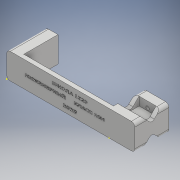
# Autodesk Inventor part: Сбрасывание
Saved by Autodesk Inventor 2018 (Build 220112000, 112)
## iProperties
Created: 2023-02-08
Part Number: Сбрасывание
Material: Типовые
Document SubType Name: Modeling
Designer: exper
Density: 1 g/cm^3
Appearance: По умолчанию
Author: exper
## iProperties of the stored document Сбрасывание_3DПЕЧАТЬ.ipt
Created: 2023-02-08
Part Number: Сбрасывание_3DПЕЧАТЬ
Material: Типовые
Document SubType Name: Modeling
Designer: exper
Density: 1 g/cm^3
Appearance: По умолчанию
Author: exper
Autodesk Inventor part; units mm, degrees
ref_plane "YZ Plane" through (0, 0, 0) normal (1, 0, 0) x (0, 1, 0)
ref_plane "XZ Plane" through (0, 0, 0) normal (0, 1, 0) x (-1, 0, 0)
ref_plane "XY Plane" through (0, 0, 0) normal (0, 0, 1) x (1, 0, 0)
sketch "Эскиз1" plane through (0, 0, 0) normal (0, 0, 1) x (1, 0, 0)
  line L0 (0, 0) -> (150, 0)
  line L1 (0, 0) -> (0, 45)
  line L2 (0, 45) -> (15, 45)
  line L3 (15, 45) -> (15, 5)
  line L4 (150, 0) -> (150, 40)
  line L5 (150, 40) -> (120, 40)
  line L6 (120, 40) -> (120, 5)
  line L7 (120, 5) -> (15, 5)
  dimension "d0" = 150
  dimension "d1" = 45
  dimension "d2" = 15
  dimension "d3" = 40
  dimension "d4" = 40
  dimension "d5" = 30
  dimension "d6" = 35
  constraints: 16 end point, 4 perpendicular, 2 vertical, 1 horizontal
  measures "d0" distance of L0.start L0.end
  measures "d1" distance of L0.start L1.end
  measures "d2" distance of L1.end L2.end
  measures "d3" distance of L2.end L3.end
  measures "d4" distance of L0.end L4.end
  measures "d5" distance of L4.end L5.end
  measures "d6" distance of L5.end L6.end
extrude "Выдавливание1" add sketch "Эскиз1" along normal blind 30
sketch "Эскиз2" plane through (120, 40, 0) normal (0, 1, 0) x (1, 0, 0)
  line L0 (0, 0) -> (0, -30) projected
  point P0 (-120, 0)
  point P1 (15, -15)
  point P2 (15, -15)
  point P3 (15, -15)
  point P4 (15, -7)
  point P5 (15, -23)
  constraints: 2 coincident
hole "Отверстие1" at (135, 40, 15) at (135, 40, 7) at (135, 40, 23) direction (0, -1, 0) diameter 4 depth 20
sketch "Эскиз3" plane through (120, 5, 0) normal (-1, 0, 0) x (0, 0, 1)
  point P0 (0, -5)
sketch "Эскиз4" plane through (120, 40, 0) normal (0, 1, 0) x (1, 0, 0)
  point P0 (-120, 0)
sketch "Эскиз5" plane through (150, 0, 0) normal (1, 0, 0) x (0, 0, -1)
  line L0 (0, 30) -> (-10, 30)
  line L1 (-10, 30) -> (-10, 10)
  line L2 (-10, 10) -> (0, 10)
  line L3 (0, 40) -> (0, 5) projected
  point P0 (0, 0)
  dimension "d19" = 10
  dimension "d20" = 20
  constraints: 6 end point, 1 horizontal, 1 perpendicular, 1 point on line, 1 vertical
  measures "d19" distance of L0.start L0.end
  measures "d20" distance of L0.end L1.end
extrude "Выдавливание2" cut sketch "Эскиз5" against normal blind 30
sketch "Эскиз6" plane through (150, 0, 30) normal (1, 0, 0) x (0, 0, -1)
  line L0 (0, 30) -> (10, 30)
  line L1 (10, 30) -> (10, 10)
  line L2 (10, 10) -> (0, 10)
  line L3 (0, 30) -> (0, 10)
  line L4 (0, 0) -> (0, 40) projected
  point P0 (30, 0)
  dimension "d24" = 10
  constraints: 8 end point, 2 perpendicular, 1 collinear, 1 horizontal
  measures "d24" distance of L0.start L0.end
extrude "Выдавливание3" cut sketch "Эскиз6" against normal blind 30
sketch "Эскиз7" plane through (150, 0, 30) normal (1, 0, 0) x (0, 0, -1)
  line L0 (30, 30) -> (20, 30) projected
  line L1 (30, 30) -> (20, 20)
  line L2 (20, 30) -> (20, 10) projected
  line L3 (30, 10) -> (30, 5) projected
  line L4 (20, 20) -> (30, 10)
  line L5 (30, 10) -> (20, 10)
  line L6 (0, 45) -> (0, 0) projected
  line L7 (20, 20) -> (20, 30)
  point P0 (30, 0)
  constraints: 8 end point, 2 perpendicular, 1 midpoint
extrude "Выдавливание4" add sketch "Эскиз7" against normal blind 5
sketch "Эскиз8" plane through (150, 0, 30) normal (1, 0, 0) x (0, 0, -1)
  line L0 (0, 30) -> (10, 30) projected
  line L1 (0, 30) -> (10, 20)
  line L2 (10, 30) -> (10, 10) projected
  line L3 (10, 10) -> (0, 10) projected
  line L4 (0, 10) -> (10, 20)
  line L5 (10, 10) -> (10, 20)
  line L6 (10, 30) -> (0, 30)
  point P0 (30, 0)
  constraints: 8 end point, 2 perpendicular, 1 midpoint, 1 point on line, 1 vertical
extrude "Выдавливание5" add sketch "Эскиз8" against normal blind 5
sketch "Эскиз9" plane through (120, 40, 0) normal (-1, 0, 0) x (0, 0, 1)
  line L0 (0, -10) -> (10, -10) projected
  line L1 (0, -10) -> (10, -20)
  line L2 (10, -10) -> (10, -30) projected
  line L3 (10, -30) -> (0, -30) projected
  line L4 (0, -30) -> (10, -20)
  line L5 (10, -30) -> (10, -20)
  line L6 (10, -10) -> (0, -10)
  point P0 (0, -40)
  constraints: 8 end point, 2 perpendicular, 1 midpoint, 1 point on line, 1 vertical
extrude "Выдавливание6" add sketch "Эскиз9" against normal blind 5
sketch "Эскиз10" plane through (120, 40, 0) normal (-1, 0, 0) x (0, 0, 1)
  line L0 (30, 0) -> (30, -10) projected
  line L1 (30, -10) -> (20, -20)
  line L2 (20, -30) -> (20, -10) projected
  line L3 (30, -30) -> (20, -30) projected
  line L4 (30, -30) -> (20, -20)
  line L5 (20, -30) -> (20, -20)
  line L6 (20, -10) -> (30, -10) projected
  line L7 (20, -10) -> (30, -10)
  point P0 (0, -40)
  constraints: 8 end point, 1 collinear, 1 midpoint, 1 perpendicular, 1 point on line, 1 vertical
extrude "Выдавливание7" add sketch "Эскиз10" against normal blind 5 contours L4 L3 L2
sketch "Эскиз11" plane through (120, 40, 0) normal (-1, 0, 0) x (0, 0, 1)
  line L0 (20, -10) -> (30, -10) projected
  line L1 (30, -10) -> (20, -20)
  line L2 (20, -20) -> (20, -10) projected
  line L3 (20, -20) -> (20, -10)
  line L4 (20, -10) -> (30, -10)
  point P0 (0, -40)
  constraints: 6 end point, 1 collinear, 1 perpendicular
extrude "Выдавливание8" add sketch "Эскиз11" against normal blind 5
sketch "Эскиз12" plane through (0, 0, 0) normal (0, -1, 0) x (1, 0, 0)
  line L0 (52.9376, 24.6029) -> (106.7977, 24.6029) construction
  line L1 (106.7977, 24.6029) -> (106.7977, 18.3352) construction
  line L2 (106.7977, 18.3352) -> (52.9376, 18.3352) construction
  line L3 (52.9376, 18.3352) -> (52.9376, 24.6029) construction
  line L4 (21.416, 17.5304) -> (72.5083, 17.5304) construction
  line L5 (72.5083, 17.5304) -> (72.5083, 13.5043) construction
  line L6 (72.5083, 13.5043) -> (21.416, 13.5043) construction
  line L7 (21.416, 13.5043) -> (21.416, 17.5304) construction
  line L8 (78.5854, 16.8541) -> (114.6972, 16.8541) construction
  line L9 (114.6972, 16.8541) -> (114.6972, 13.7301) construction
  line L10 (114.6972, 13.7301) -> (78.5854, 13.7301) construction
  line L11 (78.5854, 13.7301) -> (78.5854, 16.8541) construction
  line L12 (25.7653, 13.5409) -> (24.6543, 13.5409)
  line L13 (24.6543, 13.5409) -> (24.6543, 15.5174)
  line L14 (24.6543, 15.5174) -> (22.9258, 13.5409)
  line L15 (22.9258, 13.5409) -> (21.8804, 13.5409)
  line L16 (21.8804, 13.5409) -> (21.8804, 16.5409)
  line L17 (21.8804, 16.5409) -> (22.9914, 16.5409)
  line L18 (22.9914, 16.5409) -> (22.9914, 14.7541)
  line L19 (22.9914, 14.7541) -> (24.5911, 16.5409)
  line L20 (24.5911, 16.5409) -> (25.7653, 16.5409)
  line L21 (25.7653, 16.5409) -> (25.7653, 13.5409)
  line L22 (30.4768, 13.5409) -> (29.3464, 13.5409)
  line L23 (29.3464, 13.5409) -> (29.3464, 14.8708)
  line L24 (29.3464, 14.8708) -> (27.8075, 14.8708)
  line L25 (27.8075, 14.8708) -> (27.8075, 13.5409)
  line L26 (27.8075, 13.5409) -> (26.677, 13.5409)
  line L27 (26.677, 13.5409) -> (26.677, 16.5409)
  line L28 (26.677, 16.5409) -> (27.8075, 16.5409)
  line L29 (27.8075, 16.5409) -> (27.8075, 15.4421)
  line L30 (27.8075, 15.4421) -> (29.3464, 15.4421)
  line L31 (29.3464, 15.4421) -> (29.3464, 16.5409)
  line L32 (29.3464, 16.5409) -> (30.4768, 16.5409)
  line L33 (30.4768, 16.5409) -> (30.4768, 13.5409)
  line L34 (37.4517, 13.5409) -> (36.1219, 13.5409)
  line L35 (36.1219, 13.5409) -> (35.023, 14.7735)
  line L36 (35.023, 14.7735) -> (34.7289, 14.7735)
  line L37 (34.7289, 14.7735) -> (34.7289, 13.5409)
  line L38 (34.7289, 13.5409) -> (33.6057, 13.5409)
  line L39 (33.6057, 13.5409) -> (33.6057, 14.7735)
  line L40 (33.6057, 14.7735) -> (33.2994, 14.7735)
  line L41 (33.2994, 14.7735) -> (32.2005, 13.5409)
  line L42 (32.2005, 13.5409) -> (30.8828, 13.5409)
  line L43 (30.8828, 13.5409) -> (32.2904, 15.0701)
  spline S0 degree 2 poles (32.2904, 15.0701) (32.1859, 15.1114) (31.9987, 15.3108) (31.9015, 15.4907) knots 0 0 0 1 2 2 2
  spline S1 degree 2 poles (31.9015, 15.4907) (31.7872, 15.7095) (31.5173, 15.8894) (31.3083, 15.8894) knots 0 0 0 1 2 2 2
  line L44 (31.3083, 15.8894) -> (31.1041, 15.8894)
  line L45 (31.1041, 15.8894) -> (31.1041, 16.5409)
  spline S2 degree 2 poles (31.1041, 16.5409) (31.1575, 16.5409) (31.3812, 16.5458) (31.5246, 16.5458) knots 0 0 0 1 2 2 2
  spline S3 degree 2 poles (31.5246, 16.5458) (31.9841, 16.5458) (32.5384, 16.3075) (32.711, 16.0426) knots 0 0 0 1 2 2 2
  spline S4 degree 2 poles (32.711, 16.0426) (32.7645, 15.9599) (32.8593, 15.78) (32.9177, 15.6973) knots 0 0 0 1 2 2 2
  spline S5 degree 2 poles (32.9177, 15.6973) (33.0806, 15.4591) (33.3674, 15.2962) (33.6057, 15.2962) knots 0 0 0 1 2 2 2
  line L46 (33.6057, 15.2962) -> (33.6057, 16.5409)
  line L47 (33.6057, 16.5409) -> (34.7289, 16.5409)
  line L48 (34.7289, 16.5409) -> (34.7289, 15.2962)
  spline S6 degree 2 poles (34.7289, 15.2962) (34.9865, 15.2986) (35.2515, 15.4518) (35.4169, 15.6973) knots 0 0 0 1 2 2 2
  spline S7 degree 2 poles (35.4169, 15.6973) (35.4655, 15.7727) (35.5749, 15.9648) (35.6235, 16.0426) knots 0 0 0 1 2 2 2
  spline S8 degree 2 poles (35.6235, 16.0426) (35.7912, 16.3075) (36.348, 16.5458) (36.8099, 16.5458) knots 0 0 0 1 2 2 2
  spline S9 degree 2 poles (36.8099, 16.5458) (36.9655, 16.5458) (37.1721, 16.5409) (37.2305, 16.5409) knots 0 0 0 1 2 2 2
  line L49 (37.2305, 16.5409) -> (37.2305, 15.8967)
  line L50 (37.2305, 15.8967) -> (37.0263, 15.8967)
  spline S10 degree 2 poles (37.0263, 15.8967) (36.7783, 15.8967) (36.5571, 15.7216) (36.4233, 15.5028) knots 0 0 0 1 2 2 2
  spline S11 degree 2 poles (36.4233, 15.5028) (36.3091, 15.3108) (36.1438, 15.1212) (36.0344, 15.0774) knots 0 0 0 1 2 2 2
  line L51 (36.0344, 15.0774) -> (37.4517, 13.5409)
  line L52 (37.8601, 13.5409) -> (37.8601, 16.5409)
  line L53 (37.8601, 16.5409) -> (40.9039, 16.5409)
  line L54 (40.9039, 16.5409) -> (40.9039, 15.9696)
  line L55 (40.9039, 15.9696) -> (38.9833, 15.9696)
  line L56 (38.9833, 15.9696) -> (38.9833, 15.4421)
  line L57 (38.9833, 15.4421) -> (40.7532, 15.4421)
  line L58 (40.7532, 15.4421) -> (40.7532, 14.8708)
  line L59 (40.7532, 14.8708) -> (38.9833, 14.8708)
  line L60 (38.9833, 14.8708) -> (38.9833, 14.1122)
  line L61 (38.9833, 14.1122) -> (40.9039, 14.1122)
  line L62 (40.9039, 14.1122) -> (40.9039, 13.5409)
  line L63 (40.9039, 13.5409) -> (37.8601, 13.5409)
  line L64 (45.4671, 13.5409) -> (44.3366, 13.5409)
  line L65 (44.3366, 13.5409) -> (44.3366, 14.8708)
  line L66 (44.3366, 14.8708) -> (42.7977, 14.8708)
  line L67 (42.7977, 14.8708) -> (42.7977, 13.5409)
  line L68 (42.7977, 13.5409) -> (41.6673, 13.5409)
  line L69 (41.6673, 13.5409) -> (41.6673, 16.5409)
  line L70 (41.6673, 16.5409) -> (42.7977, 16.5409)
  line L71 (42.7977, 16.5409) -> (42.7977, 15.4421)
  line L72 (42.7977, 15.4421) -> (44.3366, 15.4421)
  line L73 (44.3366, 15.4421) -> (44.3366, 16.5409)
  line L74 (44.3366, 16.5409) -> (45.4671, 16.5409)
  line L75 (45.4671, 16.5409) -> (45.4671, 13.5409)
  line L76 (46.3934, 13.5409) -> (46.3934, 16.5409)
  line L77 (46.3934, 16.5409) -> (49.4371, 16.5409)
  line L78 (49.4371, 16.5409) -> (49.4371, 15.9696)
  line L79 (49.4371, 15.9696) -> (47.5165, 15.9696)
  line L80 (47.5165, 15.9696) -> (47.5165, 15.4421)
  line L81 (47.5165, 15.4421) -> (49.2864, 15.4421)
  line L82 (49.2864, 15.4421) -> (49.2864, 14.8708)
  line L83 (49.2864, 14.8708) -> (47.5165, 14.8708)
  line L84 (47.5165, 14.8708) -> (47.5165, 14.1122)
  line L85 (47.5165, 14.1122) -> (49.4371, 14.1122)
  line L86 (49.4371, 14.1122) -> (49.4371, 13.5409)
  line L87 (49.4371, 13.5409) -> (46.3934, 13.5409)
  spline S12 degree 2 poles (53.6648, 15.5952) (53.6648, 15.3861) (53.4655, 15.0069) (53.2783, 14.8805) knots 0 0 0 1 2 2 2
  spline S13 degree 2 poles (53.2783, 14.8805) (53.164, 14.8003) (52.8869, 14.669) (52.7216, 14.6228) knots 0 0 0 1 2 2 2
  spline S14 degree 2 poles (52.7216, 14.6228) (52.5562, 14.5766) (52.1648, 14.5231) (51.9242, 14.5231) knots 0 0 0 1 2 2 2
  line L88 (51.9242, 14.5231) -> (51.331, 14.5231)
  line L89 (51.331, 14.5231) -> (51.331, 13.5409)
  line L90 (51.331, 13.5409) -> (50.2005, 13.5409)
  line L91 (50.2005, 13.5409) -> (50.2005, 16.5409)
  line L92 (50.2005, 16.5409) -> (51.9485, 16.5409)
  spline S15 degree 2 poles (51.9485, 16.5409) (52.3374, 16.5409) (52.9039, 16.4461) (53.1324, 16.344) knots 0 0 0 1 2 2 2
  spline S16 degree 2 poles (53.1324, 16.344) (53.3877, 16.2297) (53.6648, 15.8554) (53.6648, 15.5952) knots 0 0 0 1 2 2 2
  spline S17 degree 2 poles (52.5052, 15.5758) (52.5052, 15.7046) (52.3229, 15.887) (52.1964, 15.921) knots 0 0 0 1 2 2 2
  spline S18 degree 2 poles (52.1964, 15.921) (52.036, 15.9672) (51.7418, 15.9818) (51.4914, 15.9818) knots 0 0 0 1 2 2 2
  line L93 (51.4914, 15.9818) -> (51.331, 15.9818)
  line L94 (51.331, 15.9818) -> (51.331, 15.0823)
  line L95 (51.331, 15.0823) -> (51.4088, 15.0823)
  spline S19 degree 2 poles (51.4088, 15.0823) (51.5692, 15.0823) (51.8536, 15.0871) (51.9606, 15.0993) knots 0 0 0 1 2 2 2
  spline S20 degree 2 poles (51.9606, 15.0993) (52.0506, 15.109) (52.2548, 15.1673) (52.3083, 15.2038) knots 0 0 0 1 2 2 2
  spline S21 degree 2 poles (52.3083, 15.2038) (52.4225, 15.2767) (52.5052, 15.4396) (52.5052, 15.5758) knots 0 0 0 1 2 2 2
  line L96 (58.0652, 13.5409) -> (56.9347, 13.5409)
  line L97 (56.9347, 13.5409) -> (56.9347, 14.8708)
  line L98 (56.9347, 14.8708) -> (55.3958, 14.8708)
  line L99 (55.3958, 14.8708) -> (55.3958, 13.5409)
  line L100 (55.3958, 13.5409) -> (54.2653, 13.5409)
  line L101 (54.2653, 13.5409) -> (54.2653, 16.5409)
  line L102 (54.2653, 16.5409) -> (55.3958, 16.5409)
  line L103 (55.3958, 16.5409) -> (55.3958, 15.4421)
  line L104 (55.3958, 15.4421) -> (56.9347, 15.4421)
  line L105 (56.9347, 15.4421) -> (56.9347, 16.5409)
  line L106 (56.9347, 16.5409) -> (58.0652, 16.5409)
  line L107 (58.0652, 16.5409) -> (58.0652, 13.5409)
  spline S22 degree 2 poles (62.5384, 14.5012) (62.5384, 14.28) (62.288, 13.9129) (62.0692, 13.7938) knots 0 0 0 1 2 2 2
  spline S23 degree 2 poles (62.0692, 13.7938) (61.8115, 13.6552) (61.2086, 13.5409) (60.7759, 13.5409) knots 0 0 0 1 2 2 2
  line L108 (60.7759, 13.5409) -> (58.9914, 13.5409)
  line L109 (58.9914, 13.5409) -> (58.9914, 16.5409)
  line L110 (58.9914, 16.5409) -> (60.1195, 16.5409)
  line L111 (60.1195, 16.5409) -> (60.1195, 15.4153)
  line L112 (60.1195, 15.4153) -> (60.7953, 15.4153)
  spline S24 degree 2 poles (60.7953, 15.4153) (61.1916, 15.4153) (61.831, 15.34) (62.0935, 15.2038) knots 0 0 0 1 2 2 2
  spline S25 degree 2 poles (62.0935, 15.2038) (62.3269, 15.0823) (62.5384, 14.7176) (62.5384, 14.5012) knots 0 0 0 1 2 2 2
  line L113 (64.0044, 13.5409) -> (62.8739, 13.5409)
  line L114 (62.8739, 13.5409) -> (62.8739, 16.5409)
  line L115 (62.8739, 16.5409) -> (64.0044, 16.5409)
  line L116 (64.0044, 16.5409) -> (64.0044, 13.5409)
  spline S26 degree 2 poles (61.3715, 14.4793) (61.3715, 14.5523) (61.3229, 14.686) (61.2426, 14.7419) knots 0 0 0 1 2 2 2
  spline S27 degree 2 poles (61.2426, 14.7419) (61.16, 14.7978) (60.8755, 14.861) (60.6251, 14.861) knots 0 0 0 1 2 2 2
  line L117 (60.6251, 14.861) -> (60.1195, 14.861)
  line L118 (60.1195, 14.861) -> (60.1195, 14.0977)
  line L119 (60.1195, 14.0977) -> (60.6251, 14.0977)
  spline S28 degree 2 poles (60.6251, 14.0977) (60.9703, 14.0977) (61.3715, 14.2921) (61.3715, 14.4793) knots 0 0 0 1 2 2 2
  line L120 (68.818, 13.5409) -> (67.707, 13.5409)
  line L121 (67.707, 13.5409) -> (67.707, 15.5174)
  line L122 (67.707, 15.5174) -> (65.9784, 13.5409)
  line L123 (65.9784, 13.5409) -> (64.9331, 13.5409)
  line L124 (64.9331, 13.5409) -> (64.9331, 16.5409)
  line L125 (64.9331, 16.5409) -> (66.0441, 16.5409)
  line L126 (66.0441, 16.5409) -> (66.0441, 14.7541)
  line L127 (66.0441, 14.7541) -> (67.6438, 16.5409)
  line L128 (67.6438, 16.5409) -> (68.818, 16.5409)
  line L129 (68.818, 16.5409) -> (68.818, 13.5409)
  spline S29 degree 2 poles (68.4776, 17.5304) (68.4752, 17.1682) (67.6972, 16.733) (66.8828, 16.733) knots 0 0 0 1 2 2 2
  spline S30 degree 2 poles (66.8828, 16.733) (66.0806, 16.733) (65.288, 17.173) (65.2856, 17.5304) knots 0 0 0 1 2 2 2
  line L130 (65.2856, 17.5304) -> (66.2775, 17.5304)
  spline S31 degree 2 poles (66.2775, 17.5304) (66.2823, 17.3116) (66.5498, 17.1122) (66.8828, 17.1122) knots 0 0 0 1 2 2 2
  spline S32 degree 2 poles (66.8828, 17.1122) (67.2135, 17.1122) (67.4809, 17.314) (67.4857, 17.5304) knots 0 0 0 1 2 2 2
  line L131 (67.4857, 17.5304) -> (68.4776, 17.5304)
  line L132 (53.5096, 24.5589) -> (54.3074, 24.5589)
  line L133 (54.3074, 24.5589) -> (54.369, 24.5149)
  line L134 (54.369, 24.5149) -> (54.369, 21.8781)
  line L135 (54.369, 21.8781) -> (55.8032, 21.8781)
  line L136 (55.8032, 21.8781) -> (55.8032, 24.5149)
  line L137 (55.8032, 24.5149) -> (55.8678, 24.5589)
  line L138 (55.8678, 24.5589) -> (56.6568, 24.5589)
  line L139 (56.6568, 24.5589) -> (56.7184, 24.5149)
  line L140 (56.7184, 24.5149) -> (56.7184, 21.8781)
  line L141 (56.7184, 21.8781) -> (58.1263, 21.8781)
  line L142 (58.1263, 21.8781) -> (58.1263, 24.5149)
  line L143 (58.1263, 24.5149) -> (58.1908, 24.5589)
  line L144 (58.1908, 24.5589) -> (58.9798, 24.5589)
  line L145 (58.9798, 24.5589) -> (59.0414, 24.5149)
  line L146 (59.0414, 24.5149) -> (59.0414, 21.4029)
  line L147 (59.0414, 21.4029) -> (58.9798, 21.3589)
  line L148 (58.9798, 21.3589) -> (53.5096, 21.3589)
  line L149 (53.5096, 21.3589) -> (53.4538, 21.4029)
  line L150 (53.4538, 21.4029) -> (53.4538, 24.5149)
  line L151 (53.4538, 24.5149) -> (53.5096, 24.5589)
  line L152 (60.9831, 23.2508) -> (61.467, 23.2508)
  line L153 (61.467, 23.2508) -> (62.6139, 24.5589)
  line L154 (62.6139, 24.5589) -> (63.5437, 24.5589)
  line L155 (63.5437, 24.5589) -> (63.5906, 24.5149)
  line L156 (63.5906, 24.5149) -> (62.2032, 23.0337)
  line L157 (62.2032, 23.0337) -> (63.705, 21.4029)
  line L158 (63.705, 21.4029) -> (63.661, 21.3589)
  line L159 (63.661, 21.3589) -> (62.6755, 21.3589)
  line L160 (62.6755, 21.3589) -> (61.4876, 22.7316)
  line L161 (61.4876, 22.7316) -> (60.9831, 22.7316)
  line L162 (60.9831, 22.7316) -> (60.9831, 21.4029)
  line L163 (60.9831, 21.4029) -> (60.9156, 21.3589)
  line L164 (60.9156, 21.3589) -> (60.1384, 21.3589)
  line L165 (60.1384, 21.3589) -> (60.068, 21.4029)
  line L166 (60.068, 21.4029) -> (60.068, 24.5149)
  line L167 (60.068, 24.5149) -> (60.1384, 24.5589)
  line L168 (60.1384, 24.5589) -> (60.9156, 24.5589)
  line L169 (60.9156, 24.5589) -> (60.9831, 24.5149)
  line L170 (60.9831, 24.5149) -> (60.9831, 23.2508)
  spline S33 degree 2 poles (64.0335, 22.9956) (64.0335, 23.3505) (64.2828, 23.943) (64.799, 24.3683) (65.5998, 24.6029) (66.1512, 24.6029) knots 0 0 0 1 2 3 4 4 4
  line L171 (66.1512, 24.6029) -> (66.2538, 24.6029)
  spline S34 degree 2 poles (66.2538, 24.6029) (66.8053, 24.6029) (67.6089, 24.3683) (68.1252, 23.943) (68.3745, 23.3505) (68.3745, 22.9956) knots 0 0 0 1 2 3 4 4 4
  line L172 (68.3745, 22.9956) -> (68.3745, 22.9076)
  spline S35 degree 2 poles (68.3745, 22.9076) (68.3745, 22.5498) (68.1252, 21.9631) (67.6089, 21.5466) (66.8053, 21.3149) (66.2538, 21.3149) knots 0 0 0 1 2 3 4 4 4
  line L173 (66.2538, 21.3149) -> (66.1512, 21.3149)
  spline S36 degree 2 poles (66.1512, 21.3149) (65.5998, 21.3149) (64.799, 21.5466) (64.2828, 21.9631) (64.0335, 22.5498) (64.0335, 22.9076) knots 0 0 0 1 2 3 4 4 4
  line L174 (64.0335, 22.9076) -> (64.0335, 22.9956)
  spline S37 degree 2 poles (66.1512, 24.0926) (65.8051, 24.0926) (65.3593, 23.94) (65.0923, 23.6555) (64.9867, 23.2478) (64.9867, 22.9956) knots 0 0 0 1 2 3 4 4 4
  line L175 (64.9867, 22.9956) -> (64.9867, 22.9076)
  spline S38 degree 2 poles (64.9867, 22.9076) (64.9867, 22.6553) (65.0923, 22.2564) (65.3593, 21.9749) (65.8051, 21.8253) (66.1512, 21.8253) knots 0 0 0 1 2 3 4 4 4
  line L176 (66.1512, 21.8253) -> (66.2538, 21.8253)
  spline S39 degree 2 poles (66.2538, 21.8253) (66.5999, 21.8253) (67.0487, 21.9749) (67.3127, 22.2564) (67.4153, 22.6553) (67.4153, 22.9076) knots 0 0 0 1 2 3 4 4 4
  line L177 (67.4153, 22.9076) -> (67.4153, 22.9956)
  spline S40 degree 2 poles (67.4153, 22.9956) (67.4153, 23.2478) (67.3127, 23.6555) (67.0487, 23.94) (66.5999, 24.0926) (66.2538, 24.0926) knots 0 0 0 1 2 3 4 4 4
  line L178 (66.2538, 24.0926) -> (66.1512, 24.0926)
  line L179 (72.824, 21.4029) -> (72.7506, 21.3589)
  line L180 (72.7506, 21.3589) -> (71.9763, 21.3589)
  line L181 (71.9763, 21.3589) -> (71.9059, 21.4029)
  line L182 (71.9059, 21.4029) -> (71.9059, 24.0398)
  line L183 (71.9059, 24.0398) -> (70.6447, 24.0398)
  line L184 (70.6447, 24.0398) -> (70.6447, 23.899)
  spline S41 degree 2 poles (70.6447, 23.899) (70.6447, 23.2244) (70.5713, 22.2535) (70.3132, 21.6288) (69.8234, 21.3325) (69.4098, 21.3325) knots 0 0 0 1 2 3 4 4 4
  spline S42 degree 2 poles (69.4098, 21.3325) (69.2837, 21.3325) (69.0989, 21.3355) (68.9611, 21.3413) (68.8438, 21.3531) (68.7822, 21.3619) knots 0 0 0 1 2 3 4 4 4
  line L185 (68.7822, 21.3619) -> (68.7206, 21.4117)
  line L186 (68.7206, 21.4117) -> (68.7206, 21.8194)
  line L187 (68.7206, 21.8194) -> (68.8115, 21.8634)
  spline S43 degree 2 poles (68.8115, 21.8634) (68.8848, 21.8517) (69.0491, 21.8458) (69.1341, 21.8458) knots 0 0 0 1 2 2 2
  spline S44 degree 2 poles (69.1341, 21.8458) (69.2397, 21.8458) (69.4186, 21.9045) (69.5536, 22.0629) (69.6562, 22.3474) (69.7208, 22.8049) (69.753, 23.4531) (69.753, 23.899) knots 0 0 0 1 2 3 4 5 6 6 6
  line L188 (69.753, 23.899) -> (69.753, 24.5149)
  line L189 (69.753, 24.5149) -> (69.8234, 24.5589)
  line L190 (69.8234, 24.5589) -> (72.7506, 24.5589)
  line L191 (72.7506, 24.5589) -> (72.824, 24.5149)
  line L192 (72.824, 24.5149) -> (72.824, 21.4029)
  line L193 (73.4311, 21.3589) -> (73.3871, 21.4058)
  line L194 (73.3871, 21.4058) -> (74.9886, 24.512)
  line L195 (74.9886, 24.512) -> (75.059, 24.5589)
  line L196 (75.059, 24.5589) -> (76.0914, 24.5589)
  line L197 (76.0914, 24.5589) -> (76.1618, 24.512)
  line L198 (76.1618, 24.512) -> (77.7633, 21.4058)
  line L199 (77.7633, 21.4058) -> (77.7193, 21.3589)
  line L200 (77.7193, 21.3589) -> (76.8247, 21.3589)
  line L201 (76.8247, 21.3589) -> (76.4669, 22.0629)
  line L202 (76.4669, 22.0629) -> (74.6483, 22.0629)
  line L203 (74.6483, 22.0629) -> (74.2905, 21.3589)
  line L204 (74.2905, 21.3589) -> (73.4311, 21.3589)
  line L205 (74.9153, 22.582) -> (76.1999, 22.582)
  line L206 (76.1999, 22.582) -> (75.5693, 23.9078)
  line L207 (75.5693, 23.9078) -> (75.5459, 23.9078)
  line L208 (75.5459, 23.9078) -> (74.9153, 22.582)
  line L209 (81.0366, 21.8781) -> (81.0366, 24.0456)
  line L210 (81.0366, 24.0456) -> (80.2799, 23.9371)
  line L211 (80.2799, 23.9371) -> (80.2065, 23.9694)
  line L212 (80.2065, 23.9694) -> (80.1186, 24.3712)
  line L213 (80.1186, 24.3712) -> (80.1655, 24.424)
  line L214 (80.1655, 24.424) -> (81.1393, 24.6029)
  line L215 (81.1393, 24.6029) -> (81.896, 24.6029)
  line L216 (81.896, 24.6029) -> (81.9576, 24.5589)
  line L217 (81.9576, 24.5589) -> (81.9576, 21.8781)
  line L218 (81.9576, 21.8781) -> (82.8199, 21.8781)
  line L219 (82.8199, 21.8781) -> (82.8815, 21.8341)
  line L220 (82.8815, 21.8341) -> (82.8815, 21.4029)
  line L221 (82.8815, 21.4029) -> (82.8199, 21.3589)
  line L222 (82.8199, 21.3589) -> (80.1362, 21.3589)
  line L223 (80.1362, 21.3589) -> (80.0746, 21.4029)
  line L224 (80.0746, 21.4029) -> (80.0746, 21.8341)
  line L225 (80.0746, 21.8341) -> (80.1362, 21.8781)
  line L226 (80.1362, 21.8781) -> (81.0366, 21.8781)
  line L227 (83.6559, 24.0838) -> (83.6559, 24.5149)
  line L228 (83.6559, 24.5149) -> (83.7175, 24.5589)
  line L229 (83.7175, 24.5589) -> (86.325, 24.5589)
  line L230 (86.325, 24.5589) -> (86.3866, 24.5149)
  line L231 (86.3866, 24.5149) -> (86.3866, 24.0574)
  line L232 (86.3866, 24.0574) -> (85.4568, 23.2097)
  spline S45 degree 2 poles (85.4568, 23.2097) (85.7296, 23.1745) (86.1754, 23.0454) (86.4863, 22.8372) (86.6564, 22.541) (86.6564, 22.3356) knots 0 0 0 1 2 3 4 4 4
  line L233 (86.6564, 22.3356) -> (86.6564, 22.2916)
  spline S46 degree 2 poles (86.6564, 22.2916) (86.6564, 22.0482) (86.413, 21.6786) (85.9759, 21.4381) (85.3629, 21.3149) (84.9963, 21.3149) knots 0 0 0 1 2 3 4 4 4
  line L234 (84.9963, 21.3149) -> (84.9054, 21.3149)
  spline S47 degree 2 poles (84.9054, 21.3149) (84.7646, 21.3149) (84.4507, 21.3355) (84.1281, 21.3736) (83.7996, 21.4176) (83.6471, 21.444) knots 0 0 0 1 2 3 4 4 4
  line L235 (83.6471, 21.444) -> (83.5825, 21.4968)
  line L236 (83.5825, 21.4968) -> (83.5825, 21.9631)
  line L237 (83.5825, 21.9631) -> (83.6441, 22.0071)
  line L238 (83.6441, 22.0071) -> (83.6735, 22.0071)
  spline S48 degree 2 poles (83.6735, 22.0071) (83.8054, 21.9719) (84.0548, 21.9133) (84.307, 21.8693) (84.571, 21.8487) (84.7176, 21.8487) knots 0 0 0 1 2 3 4 4 4
  line L239 (84.7176, 21.8487) -> (84.8086, 21.8487)
  spline S49 degree 2 poles (84.8086, 21.8487) (85.2573, 21.8487) (85.7354, 22.0834) (85.7354, 22.2916) knots 0 0 0 1 2 2 2
  line L240 (85.7354, 22.2916) -> (85.7354, 22.3356)
  spline S50 degree 2 poles (85.7354, 22.3356) (85.7354, 22.5322) (85.2573, 22.7433) (84.7323, 22.7433) knots 0 0 0 1 2 2 2
  line L241 (84.7323, 22.7433) -> (84.6032, 22.7433)
  line L242 (84.6032, 22.7433) -> (84.4155, 23.1364)
  line L243 (84.4155, 23.1364) -> (85.3834, 24.0398)
  line L244 (85.3834, 24.0398) -> (83.7175, 24.0398)
  line L245 (83.7175, 24.0398) -> (83.6559, 24.0838)
  line L246 (87.2606, 21.8927) -> (88.2373, 22.5879)
  spline S51 degree 2 poles (88.2373, 22.5879) (88.5629, 22.8167) (88.9794, 23.1364) (89.2258, 23.3739) (89.3226, 23.5587) (89.3226, 23.6555) knots 0 0 0 1 2 3 4 4 4
  line L247 (89.3226, 23.6555) -> (89.3226, 23.7201)
  spline S52 degree 2 poles (89.3226, 23.7201) (89.3226, 23.7934) (89.2551, 23.9166) (89.1026, 24.0134) (88.8621, 24.0691) (88.689, 24.0691) knots 0 0 0 1 2 3 4 4 4
  line L248 (88.689, 24.0691) -> (88.5952, 24.0691)
  spline S53 degree 2 poles (88.5952, 24.0691) (88.3664, 24.0691) (87.8414, 23.984) (87.5715, 23.8814) knots 0 0 0 1 2 2 2
  line L249 (87.5715, 23.8814) -> (87.4865, 23.9166)
  line L250 (87.4865, 23.9166) -> (87.4014, 24.3741)
  line L251 (87.4014, 24.3741) -> (87.4571, 24.424)
  spline S54 degree 2 poles (87.4571, 24.424) (87.5921, 24.4621) (87.9147, 24.5296) (88.2403, 24.5765) (88.5629, 24.6029) (88.7037, 24.6029) knots 0 0 0 1 2 3 4 4 4
  line L252 (88.7037, 24.6029) -> (88.7976, 24.6029)
  spline S55 degree 2 poles (88.7976, 24.6029) (89.1026, 24.6029) (89.6335, 24.4915) (90.0265, 24.2656) (90.2494, 23.9371) (90.2494, 23.7201) knots 0 0 0 1 2 3 4 4 4
  line L253 (90.2494, 23.7201) -> (90.2494, 23.6555)
  spline S56 degree 2 poles (90.2494, 23.6555) (90.2494, 23.5294) (90.1439, 23.2684) (89.8681, 22.9604) (89.3959, 22.5732) (89.0263, 22.321) knots 0 0 0 1 2 3 4 4 4
  line L254 (89.0263, 22.321) -> (88.3869, 21.8781)
  line L255 (88.3869, 21.8781) -> (90.3257, 21.8781)
  line L256 (90.3257, 21.8781) -> (90.3844, 21.8341)
  line L257 (90.3844, 21.8341) -> (90.3844, 21.4029)
  line L258 (90.3844, 21.4029) -> (90.3257, 21.3589)
  line L259 (90.3257, 21.3589) -> (87.3222, 21.3589)
  line L260 (87.3222, 21.3589) -> (87.2606, 21.4029)
  line L261 (87.2606, 21.4029) -> (87.2606, 21.8927)
  line L262 (91.2526, 21.9191) -> (91.3318, 21.9631)
  spline S57 degree 2 poles (91.3318, 21.9631) (91.4344, 21.9279) (91.6691, 21.8839) (91.8978, 21.8605) (92.1178, 21.8487) (92.2058, 21.8487) knots 0 0 0 1 2 3 4 4 4
  line L263 (92.2058, 21.8487) -> (92.2674, 21.8487)
  spline S58 degree 2 poles (92.2674, 21.8487) (92.5226, 21.8487) (92.8892, 21.969) (93.1239, 22.1919) (93.2353, 22.5116) (93.2353, 22.7111) knots 0 0 0 1 2 3 4 4 4
  line L264 (93.2353, 22.7111) -> (93.2353, 22.7551)
  spline S59 degree 2 poles (93.2353, 22.7551) (93.0271, 22.6524) (92.5783, 22.5498) (92.3965, 22.5498) knots 0 0 0 1 2 2 2
  line L265 (92.3965, 22.5498) -> (92.3319, 22.5498)
  spline S60 degree 2 poles (92.3319, 22.5498) (92.0093, 22.5498) (91.4843, 22.6788) (91.1059, 22.9252) (90.9006, 23.2772) (90.9006, 23.4971) knots 0 0 0 1 2 3 4 4 4
  line L266 (90.9006, 23.4971) -> (90.9006, 23.5822)
  spline S61 degree 2 poles (90.9006, 23.5822) (90.9006, 23.8139) (91.1382, 24.1893) (91.5605, 24.4563) (92.1354, 24.6029) (92.4786, 24.6029) knots 0 0 0 1 2 3 4 4 4
  line L267 (92.4786, 24.6029) -> (92.5431, 24.6029)
  spline S62 degree 2 poles (92.5431, 24.6029) (93.0036, 24.6029) (93.6254, 24.3917) (93.9979, 24.0134) (94.1592, 23.4883) (94.1592, 23.1745) knots 0 0 0 1 2 3 4 4 4
  line L268 (94.1592, 23.1745) -> (94.1592, 22.9193)
  spline S63 degree 2 poles (94.1592, 22.9193) (94.1592, 22.582) (93.9627, 21.9954) (93.5228, 21.5613) (92.8247, 21.3149) (92.3231, 21.3149) knots 0 0 0 1 2 3 4 4 4
  line L269 (92.3231, 21.3149) -> (92.2733, 21.3149)
  spline S64 degree 2 poles (92.2733, 21.3149) (92.1677, 21.3149) (91.9008, 21.3267) (91.6221, 21.3531) (91.3494, 21.3941) (91.2438, 21.4234) knots 0 0 0 1 2 3 4 4 4
  line L270 (91.2438, 21.4234) -> (91.188, 21.4674)
  line L271 (91.188, 21.4674) -> (91.2526, 21.9191)
  spline S65 degree 2 poles (93.2353, 23.2566) (93.2353, 23.5059) (93.1767, 23.8286) (93.0271, 24.0192) (92.7572, 24.0926) (92.5431, 24.0926) knots 0 0 0 1 2 3 4 4 4
  line L272 (92.5431, 24.0926) -> (92.4786, 24.0926)
  spline S66 degree 2 poles (92.4786, 24.0926) (92.3671, 24.0926) (92.1354, 24.0456) (91.9448, 23.9283) (91.8216, 23.7318) (91.8216, 23.5851) knots 0 0 0 1 2 3 4 4 4
  line L273 (91.8216, 23.5851) -> (91.8216, 23.4971)
  spline S67 degree 2 poles (91.8216, 23.4971) (91.8216, 23.3446) (91.9536, 23.1628) (92.1501, 23.0689) (92.3877, 23.0396) (92.4933, 23.0396) knots 0 0 0 1 2 3 4 4 4
  line L274 (92.4933, 23.0396) -> (92.5549, 23.0396)
  spline S68 degree 2 poles (92.5549, 23.0396) (92.6692, 23.0396) (93.0447, 23.1393) (93.2353, 23.2566) knots 0 0 0 1 2 2 2
  line L275 (83.0173, 13.7933) -> (81.6704, 13.7933)
  line L276 (81.6704, 13.7933) -> (80.4646, 15.004)
  line L277 (80.4646, 15.004) -> (80.1802, 15.004)
  line L278 (80.1802, 15.004) -> (80.1802, 13.7933)
  line L279 (80.1802, 13.7933) -> (79.0497, 13.7933)
  line L280 (79.0497, 13.7933) -> (79.0497, 16.7933)
  line L281 (79.0497, 16.7933) -> (80.1802, 16.7933)
  line L282 (80.1802, 16.7933) -> (80.1802, 15.5704)
  spline S69 degree 2 poles (80.1802, 15.5704) (80.4452, 15.5777) (80.7077, 15.7187) (80.8876, 15.9594) knots 0 0 0 1 2 2 2
  spline S70 degree 2 poles (80.8876, 15.9594) (80.9387, 16.0299) (81.0748, 16.222) (81.1259, 16.2949) knots 0 0 0 1 2 2 2
  spline S71 degree 2 poles (81.1259, 16.2949) (81.3228, 16.5672) (81.8892, 16.7981) (82.3512, 16.7981) knots 0 0 0 1 2 2 2
  spline S72 degree 2 poles (82.3512, 16.7981) (82.5043, 16.7981) (82.7037, 16.7933) (82.7572, 16.7933) knots 0 0 0 1 2 2 2
  line L283 (82.7572, 16.7933) -> (82.7572, 16.149)
  line L284 (82.7572, 16.149) -> (82.497, 16.149)
  spline S73 degree 2 poles (82.497, 16.149) (82.305, 16.149) (82.0181, 15.991) (81.8698, 15.7528) knots 0 0 0 1 2 2 2
  spline S74 degree 2 poles (81.8698, 15.7528) (81.7507, 15.5631) (81.5416, 15.3686) (81.4516, 15.3346) knots 0 0 0 1 2 2 2
  line L285 (81.4516, 15.3346) -> (83.0173, 13.7933)
  line L286 (87.2572, 13.7933) -> (86.1267, 13.7933)
  line L287 (86.1267, 13.7933) -> (86.1267, 16.222)
  line L288 (86.1267, 16.222) -> (84.9889, 16.222)
  spline S75 degree 2 poles (84.9889, 16.222) (84.9768, 16.0469) (84.9549, 15.743) (84.9427, 15.6045) knots 0 0 0 1 2 2 2
  spline S76 degree 2 poles (84.9427, 15.6045) (84.9111, 15.213) (84.7604, 14.6417) (84.6632, 14.4618) knots 0 0 0 1 2 2 2
  spline S77 degree 2 poles (84.6632, 14.4618) (84.5562, 14.2673) (84.3398, 14.0461) (84.2426, 13.9805) knots 0 0 0 1 2 2 2
  spline S78 degree 2 poles (84.2426, 13.9805) (84.0991, 13.8857) (83.664, 13.7738) (83.4525, 13.7738) knots 0 0 0 1 2 2 2
  spline S79 degree 2 poles (83.4525, 13.7738) (83.3115, 13.7738) (82.9735, 13.7908) (82.9273, 13.7933) knots 0 0 0 1 2 2 2
  line L289 (82.9273, 13.7933) -> (82.9273, 14.4545)
  line L290 (82.9273, 14.4545) -> (82.9687, 14.4545)
  spline S80 degree 2 poles (82.9687, 14.4545) (83.0003, 14.4545) (83.0562, 14.4497) (83.1024, 14.4497) knots 0 0 0 1 2 2 2
  spline S81 degree 2 poles (83.1024, 14.4497) (83.1777, 14.4497) (83.4136, 14.4813) (83.4743, 14.5202) knots 0 0 0 1 2 2 2
  spline S82 degree 2 poles (83.4743, 14.5202) (83.6907, 14.6563) (83.8512, 15.2325) (83.8925, 15.7746) knots 0 0 0 1 2 2 2
  spline S83 degree 2 poles (83.8925, 15.7746) (83.9119, 16.0226) (83.9217, 16.4164) (83.9387, 16.7933) knots 0 0 0 1 2 2 2
  line L291 (83.9387, 16.7933) -> (87.2572, 16.7933)
  line L292 (87.2572, 16.7933) -> (87.2572, 13.7933)
  line L293 (87.7045, 13.7933) -> (89.2239, 16.7933)
  line L294 (89.2239, 16.7933) -> (90.4541, 16.7933)
  line L295 (90.4541, 16.7933) -> (91.9735, 13.7933)
  line L296 (91.9735, 13.7933) -> (90.809, 13.7933)
  line L297 (90.809, 13.7933) -> (90.5294, 14.4059)
  line L298 (90.5294, 14.4059) -> (89.1194, 14.4059)
  line L299 (89.1194, 14.4059) -> (88.8374, 13.7933)
  line L300 (88.8374, 13.7933) -> (87.7045, 13.7933)
  line L301 (90.2815, 14.9505) -> (89.8244, 15.9375)
  line L302 (89.8244, 15.9375) -> (89.3674, 14.9505)
  line L303 (89.3674, 14.9505) -> (90.2815, 14.9505)
  spline S84 degree 2 poles (94.3609, 13.7349) (93.3495, 13.7349) (92.1583, 14.5518) (92.1583, 15.2908) knots 0 0 0 1 2 2 2
  spline S85 degree 2 poles (92.1583, 15.2908) (92.1583, 16.0032) (93.352, 16.8516) (94.3633, 16.8516) knots 0 0 0 1 2 2 2
  spline S86 degree 2 poles (94.3633, 16.8516) (94.6332, 16.8516) (95.0635, 16.8103) (95.258, 16.7763) knots 0 0 0 1 2 2 2
  spline S87 degree 2 poles (95.258, 16.7763) (95.4136, 16.7447) (95.7758, 16.6401) (95.8876, 16.6012) knots 0 0 0 1 2 2 2
  line L304 (95.8876, 16.6012) -> (95.8876, 15.8865)
  line L305 (95.8876, 15.8865) -> (95.7734, 15.8865)
  spline S88 degree 2 poles (95.7734, 15.8865) (95.6907, 15.9351) (95.4427, 16.0712) (95.2871, 16.1344) knots 0 0 0 1 2 2 2
  spline S89 degree 2 poles (95.2871, 16.1344) (95.1291, 16.2001) (94.7523, 16.29) (94.5457, 16.29) knots 0 0 0 1 2 2 2
  spline S90 degree 2 poles (94.5457, 16.29) (94.3001, 16.29) (93.8941, 16.1879) (93.7093, 16.0591) knots 0 0 0 1 2 2 2
  spline S91 degree 2 poles (93.7093, 16.0591) (93.5392, 15.9448) (93.3252, 15.5534) (93.3252, 15.2884) knots 0 0 0 1 2 2 2
  spline S92 degree 2 poles (93.3252, 15.2884) (93.3252, 15.0088) (93.5489, 14.6271) (93.7312, 14.5105) knots 0 0 0 1 2 2 2
  spline S93 degree 2 poles (93.7312, 14.5105) (93.9063, 14.3962) (94.3366, 14.2965) (94.5529, 14.2965) knots 0 0 0 1 2 2 2
  spline S94 degree 2 poles (94.5529, 14.2965) (94.7766, 14.2965) (95.1802, 14.3962) (95.3187, 14.457) knots 0 0 0 1 2 2 2
  spline S95 degree 2 poles (95.3187, 14.457) (95.4695, 14.5177) (95.7004, 14.6466) (95.7855, 14.6976) knots 0 0 0 1 2 2 2
  line L306 (95.7855, 14.6976) -> (95.8876, 14.6976)
  line L307 (95.8876, 14.6976) -> (95.8876, 13.9926)
  spline S96 degree 2 poles (95.8876, 13.9926) (95.7636, 13.9537) (95.4379, 13.8565) (95.2653, 13.8224) knots 0 0 0 1 2 2 2
  spline S97 degree 2 poles (95.2653, 13.8224) (95.0538, 13.7787) (94.6842, 13.7349) (94.3609, 13.7349) knots 0 0 0 1 2 2 2
  spline S98 degree 2 poles (98.4889, 13.7349) (97.4776, 13.7349) (96.2863, 14.5518) (96.2863, 15.2908) knots 0 0 0 1 2 2 2
  spline S99 degree 2 poles (96.2863, 15.2908) (96.2863, 16.0032) (97.48, 16.8516) (98.4914, 16.8516) knots 0 0 0 1 2 2 2
  spline S100 degree 2 poles (98.4914, 16.8516) (98.7612, 16.8516) (99.1915, 16.8103) (99.386, 16.7763) knots 0 0 0 1 2 2 2
  spline S101 degree 2 poles (99.386, 16.7763) (99.5416, 16.7447) (99.9038, 16.6401) (100.0157, 16.6012) knots 0 0 0 1 2 2 2
  line L308 (100.0157, 16.6012) -> (100.0157, 15.8865)
  line L309 (100.0157, 15.8865) -> (99.9014, 15.8865)
  spline S102 degree 2 poles (99.9014, 15.8865) (99.8187, 15.9351) (99.5708, 16.0712) (99.4152, 16.1344) knots 0 0 0 1 2 2 2
  spline S103 degree 2 poles (99.4152, 16.1344) (99.2572, 16.2001) (98.8803, 16.29) (98.6737, 16.29) knots 0 0 0 1 2 2 2
  spline S104 degree 2 poles (98.6737, 16.29) (98.4281, 16.29) (98.0222, 16.1879) (97.8374, 16.0591) knots 0 0 0 1 2 2 2
  spline S105 degree 2 poles (97.8374, 16.0591) (97.6672, 15.9448) (97.4533, 15.5534) (97.4533, 15.2884) knots 0 0 0 1 2 2 2
  spline S106 degree 2 poles (97.4533, 15.2884) (97.4533, 15.0088) (97.6769, 14.6271) (97.8593, 14.5105) knots 0 0 0 1 2 2 2
  spline S107 degree 2 poles (97.8593, 14.5105) (98.0343, 14.3962) (98.4646, 14.2965) (98.681, 14.2965) knots 0 0 0 1 2 2 2
  spline S108 degree 2 poles (98.681, 14.2965) (98.9046, 14.2965) (99.3082, 14.3962) (99.4468, 14.457) knots 0 0 0 1 2 2 2
  spline S109 degree 2 poles (99.4468, 14.457) (99.5975, 14.5177) (99.8285, 14.6466) (99.9136, 14.6976) knots 0 0 0 1 2 2 2
  line L310 (99.9136, 14.6976) -> (100.0157, 14.6976)
  line L311 (100.0157, 14.6976) -> (100.0157, 13.9926)
  spline S110 degree 2 poles (100.0157, 13.9926) (99.8917, 13.9537) (99.5659, 13.8565) (99.3933, 13.8224) knots 0 0 0 1 2 2 2
  spline S111 degree 2 poles (99.3933, 13.8224) (99.1818, 13.7787) (98.8123, 13.7349) (98.4889, 13.7349) knots 0 0 0 1 2 2 2
  line L312 (105.5854, 13.7933) -> (102.6121, 13.7933)
  line L313 (102.6121, 13.7933) -> (102.6121, 14.316)
  line L314 (102.6121, 14.316) -> (103.5602, 14.316)
  line L315 (103.5602, 14.316) -> (103.5602, 15.9035)
  line L316 (103.5602, 15.9035) -> (102.6121, 15.9035)
  line L317 (102.6121, 15.9035) -> (102.6121, 16.3921)
  spline S112 degree 2 poles (102.6121, 16.3921) (102.8212, 16.3921) (103.232, 16.4286) (103.356, 16.4675) knots 0 0 0 1 2 2 2
  spline S113 degree 2 poles (103.356, 16.4675) (103.4995, 16.5161) (103.6599, 16.679) (103.6721, 16.8006) knots 0 0 0 1 2 2 2
  line L318 (103.6721, 16.8006) -> (104.6567, 16.8006)
  line L319 (104.6567, 16.8006) -> (104.6567, 14.316)
  line L320 (104.6567, 14.316) -> (105.5854, 14.316)
  line L321 (105.5854, 14.316) -> (105.5854, 13.7933)
  spline S114 degree 2 poles (109.6648, 15.2933) (109.6648, 14.9043) (109.4776, 14.3208) (109.2734, 14.1239) knots 0 0 0 1 2 2 2
  spline S115 degree 2 poles (109.2734, 14.1239) (109.0667, 13.9294) (108.4079, 13.7301) (107.9314, 13.7301) knots 0 0 0 1 2 2 2
  spline S116 degree 2 poles (107.9314, 13.7301) (107.4573, 13.7301) (106.7985, 13.9294) (106.5894, 14.1288) knots 0 0 0 1 2 2 2
  spline S117 degree 2 poles (106.5894, 14.1288) (106.3852, 14.3257) (106.198, 14.9043) (106.198, 15.2933) knots 0 0 0 1 2 2 2
  spline S118 degree 2 poles (106.198, 15.2933) (106.198, 15.692) (106.3828, 16.256) (106.5967, 16.4602) knots 0 0 0 1 2 2 2
  spline S119 degree 2 poles (106.5967, 16.4602) (106.8082, 16.6596) (107.4719, 16.8541) (107.9314, 16.8541) knots 0 0 0 1 2 2 2
  spline S120 degree 2 poles (107.9314, 16.8541) (108.4176, 16.8541) (109.0667, 16.6498) (109.2758, 16.4481) knots 0 0 0 1 2 2 2
  spline S121 degree 2 poles (109.2758, 16.4481) (109.48, 16.2511) (109.6648, 15.6701) (109.6648, 15.2933) knots 0 0 0 1 2 2 2
  spline S122 degree 2 poles (108.5319, 15.2933) (108.5319, 15.85) (108.2572, 16.2998) (107.9314, 16.2998) knots 0 0 0 1 2 2 2
  spline S123 degree 2 poles (107.9314, 16.2998) (107.6081, 16.2998) (107.3309, 15.85) (107.3309, 15.2908) knots 0 0 0 1 2 2 2
  spline S124 degree 2 poles (107.3309, 15.2908) (107.3309, 14.7414) (107.6081, 14.2844) (107.9314, 14.2844) knots 0 0 0 1 2 2 2
  spline S125 degree 2 poles (107.9314, 14.2844) (108.2547, 14.2844) (108.5319, 14.7414) (108.5319, 15.2933) knots 0 0 0 1 2 2 2
  line L322 (114.2499, 13.7933) -> (113.1388, 13.7933)
  line L323 (113.1388, 13.7933) -> (113.1388, 15.7698)
  line L324 (113.1388, 15.7698) -> (111.4103, 13.7933)
  line L325 (111.4103, 13.7933) -> (110.3649, 13.7933)
  line L326 (110.3649, 13.7933) -> (110.3649, 16.7933)
  line L327 (110.3649, 16.7933) -> (111.476, 16.7933)
  line L328 (111.476, 16.7933) -> (111.476, 15.0064)
  line L329 (111.476, 15.0064) -> (113.0756, 16.7933)
  line L330 (113.0756, 16.7933) -> (114.2499, 16.7933)
  line L331 (114.2499, 16.7933) -> (114.2499, 13.7933)
  point P0 (0, 0)
  constraints: 6 other
sketch "Эскиз13" plane through (0, 0, 0) normal (0, -1, 0) x (1, 0, 0)
  point P0 (0, 0)
sketch "Эскиз14" plane through (0, 0, 0) normal (0, -1, 0) x (1, 0, 0)
  line L0 (65.4998, 8.3262) -> (82.3037, 8.3262) construction
  line L1 (82.3037, 8.3262) -> (82.3037, 4.9914) construction
  line L2 (82.3037, 4.9914) -> (65.4998, 4.9914) construction
  line L3 (65.4998, 4.9914) -> (65.4998, 8.3262) construction
  line L4 (69.5115, 5.0588) -> (65.9873, 5.0588)
  line L5 (65.9873, 5.0588) -> (65.9873, 5.5801)
  spline S0 degree 2 poles (65.9873, 5.5801) (66.4359, 5.8186) (67.1465, 6.2387) (67.4162, 6.428) knots 0 0 0 1 2 2 2
  spline S1 degree 2 poles (67.4162, 6.428) (67.7663, 6.6744) (68.0826, 7.0504) (68.0826, 7.2475) knots 0 0 0 1 2 2 2
  spline S2 degree 2 poles (68.0826, 7.2475) (68.0826, 7.4705) (67.6833, 7.7091) (67.3254, 7.7091) knots 0 0 0 1 2 2 2
  spline S3 degree 2 poles (67.3254, 7.7091) (67.1439, 7.7091) (66.8171, 7.6494) (66.6512, 7.6027) knots 0 0 0 1 2 2 2
  spline S4 degree 2 poles (66.6512, 7.6027) (66.4878, 7.5535) (66.2544, 7.4497) (66.1974, 7.4238) knots 0 0 0 1 2 2 2
  line L6 (66.1974, 7.4238) -> (66.104, 7.4238)
  line L7 (66.104, 7.4238) -> (66.104, 8.1214)
  spline S5 degree 2 poles (66.104, 8.1214) (66.3063, 8.1862) (67.1698, 8.3211) (67.5692, 8.3211) knots 0 0 0 1 2 2 2
  spline S6 degree 2 poles (67.5692, 8.3211) (68.4223, 8.3211) (69.3014, 7.8128) (69.3014, 7.3538) knots 0 0 0 1 2 2 2
  spline S7 degree 2 poles (69.3014, 7.3538) (69.3014, 7.0711) (68.9021, 6.5266) (68.4379, 6.2154) knots 0 0 0 1 2 2 2
  spline S8 degree 2 poles (68.4379, 6.2154) (68.1475, 6.0235) (67.6003, 5.7253) (67.4784, 5.663) knots 0 0 0 1 2 2 2
  line L8 (67.4784, 5.663) -> (69.5115, 5.663)
  line L9 (69.5115, 5.663) -> (69.5115, 5.0588)
  spline S9 degree 2 poles (73.6502, 6.6588) (73.6502, 6.2439) (73.4505, 5.6215) (73.2327, 5.4115) knots 0 0 0 1 2 2 2
  spline S10 degree 2 poles (73.2327, 5.4115) (73.0123, 5.204) (72.3095, 4.9914) (71.8013, 4.9914) knots 0 0 0 1 2 2 2
  spline S11 degree 2 poles (71.8013, 4.9914) (71.2956, 4.9914) (70.5928, 5.204) (70.3698, 5.4167) knots 0 0 0 1 2 2 2
  spline S12 degree 2 poles (70.3698, 5.4167) (70.152, 5.6267) (69.9523, 6.2439) (69.9523, 6.6588) knots 0 0 0 1 2 2 2
  spline S13 degree 2 poles (69.9523, 6.6588) (69.9523, 7.0841) (70.1494, 7.6857) (70.3776, 7.9036) knots 0 0 0 1 2 2 2
  spline S14 degree 2 poles (70.3776, 7.9036) (70.6032, 8.1162) (71.3111, 8.3237) (71.8013, 8.3237) knots 0 0 0 1 2 2 2
  spline S15 degree 2 poles (71.8013, 8.3237) (72.3199, 8.3237) (73.0123, 8.1058) (73.2353, 7.8906) knots 0 0 0 1 2 2 2
  spline S16 degree 2 poles (73.2353, 7.8906) (73.4531, 7.6805) (73.6502, 7.0608) (73.6502, 6.6588) knots 0 0 0 1 2 2 2
  spline S17 degree 2 poles (72.4418, 6.6588) (72.4418, 7.2527) (72.1488, 7.7324) (71.8013, 7.7324) knots 0 0 0 1 2 2 2
  spline S18 degree 2 poles (71.8013, 7.7324) (71.4564, 7.7324) (71.1607, 7.2527) (71.1607, 6.6562) knots 0 0 0 1 2 2 2
  spline S19 degree 2 poles (71.1607, 6.6562) (71.1607, 6.0702) (71.4564, 5.5826) (71.8013, 5.5826) knots 0 0 0 1 2 2 2
  spline S20 degree 2 poles (71.8013, 5.5826) (72.1462, 5.5826) (72.4418, 6.0702) (72.4418, 6.6588) knots 0 0 0 1 2 2 2
  line L10 (77.9134, 5.0588) -> (74.3893, 5.0588)
  line L11 (74.3893, 5.0588) -> (74.3893, 5.5801)
  spline S21 degree 2 poles (74.3893, 5.5801) (74.8379, 5.8186) (75.5484, 6.2387) (75.8181, 6.428) knots 0 0 0 1 2 2 2
  spline S22 degree 2 poles (75.8181, 6.428) (76.1682, 6.6744) (76.4846, 7.0504) (76.4846, 7.2475) knots 0 0 0 1 2 2 2
  spline S23 degree 2 poles (76.4846, 7.2475) (76.4846, 7.4705) (76.0852, 7.7091) (75.7274, 7.7091) knots 0 0 0 1 2 2 2
  spline S24 degree 2 poles (75.7274, 7.7091) (75.5458, 7.7091) (75.2191, 7.6494) (75.0531, 7.6027) knots 0 0 0 1 2 2 2
  spline S25 degree 2 poles (75.0531, 7.6027) (74.8898, 7.5535) (74.6564, 7.4497) (74.5993, 7.4238) knots 0 0 0 1 2 2 2
  line L12 (74.5993, 7.4238) -> (74.506, 7.4238)
  line L13 (74.506, 7.4238) -> (74.506, 8.1214)
  spline S26 degree 2 poles (74.506, 8.1214) (74.7082, 8.1862) (75.5718, 8.3211) (75.9711, 8.3211) knots 0 0 0 1 2 2 2
  spline S27 degree 2 poles (75.9711, 8.3211) (76.8243, 8.3211) (77.7034, 7.8128) (77.7034, 7.3538) knots 0 0 0 1 2 2 2
  spline S28 degree 2 poles (77.7034, 7.3538) (77.7034, 7.0711) (77.304, 6.5266) (76.8398, 6.2154) knots 0 0 0 1 2 2 2
  spline S29 degree 2 poles (76.8398, 6.2154) (76.5494, 6.0235) (76.0022, 5.7253) (75.8804, 5.663) knots 0 0 0 1 2 2 2
  line L14 (75.8804, 5.663) -> (77.9134, 5.663)
  line L15 (77.9134, 5.663) -> (77.9134, 5.0588)
  spline S30 degree 2 poles (81.9951, 6.0287) (81.9951, 5.7927) (81.7332, 5.4063) (81.4817, 5.2715) knots 0 0 0 1 2 2 2
  spline S31 degree 2 poles (81.4817, 5.2715) (81.2275, 5.1366) (80.5429, 4.9914) (80.0502, 4.9914) knots 0 0 0 1 2 2 2
  spline S32 degree 2 poles (80.0502, 4.9914) (79.4875, 4.9914) (78.6862, 5.1159) (78.4346, 5.1937) knots 0 0 0 1 2 2 2
  line L16 (78.4346, 5.1937) -> (78.4346, 5.8886)
  line L17 (78.4346, 5.8886) -> (78.5513, 5.8886)
  spline S33 degree 2 poles (78.5513, 5.8886) (78.8158, 5.7771) (79.529, 5.6112) (79.822, 5.6112) knots 0 0 0 1 2 2 2
  spline S34 degree 2 poles (79.822, 5.6112) (79.9958, 5.6112) (80.4055, 5.6527) (80.5455, 5.7201) knots 0 0 0 1 2 2 2
  spline S35 degree 2 poles (80.5455, 5.7201) (80.6544, 5.7745) (80.7867, 5.9327) (80.7867, 6.0754) knots 0 0 0 1 2 2 2
  spline S36 degree 2 poles (80.7867, 6.0754) (80.7867, 6.218) (80.6, 6.371) (80.4444, 6.4073) knots 0 0 0 1 2 2 2
  spline S37 degree 2 poles (80.4444, 6.4073) (80.2888, 6.4436) (79.8557, 6.4514) (79.6923, 6.4514) knots 0 0 0 1 2 2 2
  line L18 (79.6923, 6.4514) -> (79.4849, 6.4514)
  line L19 (79.4849, 6.4514) -> (79.4849, 7.0141)
  line L20 (79.4849, 7.0141) -> (79.6742, 7.0141)
  spline S38 degree 2 poles (79.6742, 7.0141) (79.8946, 7.0141) (80.2603, 7.04) (80.3899, 7.0789) knots 0 0 0 1 2 2 2
  spline S39 degree 2 poles (80.3899, 7.0789) (80.517, 7.1204) (80.6622, 7.2656) (80.6622, 7.3901) knots 0 0 0 1 2 2 2
  spline S40 degree 2 poles (80.6622, 7.3901) (80.6622, 7.4886) (80.5274, 7.6105) (80.4262, 7.6442) knots 0 0 0 1 2 2 2
  spline S41 degree 2 poles (80.4262, 7.6442) (80.3121, 7.6831) (80.0009, 7.7091) (79.892, 7.7091) knots 0 0 0 1 2 2 2
  spline S42 degree 2 poles (79.892, 7.7091) (79.7157, 7.7091) (79.3475, 7.6546) (79.1737, 7.6105) knots 0 0 0 1 2 2 2
  spline S43 degree 2 poles (79.1737, 7.6105) (79.0389, 7.5768) (78.7432, 7.4679) (78.6732, 7.4394) knots 0 0 0 1 2 2 2
  line L21 (78.6732, 7.4394) -> (78.5721, 7.4394)
  line L22 (78.5721, 7.4394) -> (78.5721, 8.124)
  spline S44 degree 2 poles (78.5721, 8.124) (78.821, 8.194) (79.6612, 8.3262) (80.0995, 8.3262) knots 0 0 0 1 2 2 2
  spline S45 degree 2 poles (80.0995, 8.3262) (80.5299, 8.3262) (81.1575, 8.2277) (81.3805, 8.1318) knots 0 0 0 1 2 2 2
  spline S46 degree 2 poles (81.3805, 8.1318) (81.6269, 8.0306) (81.8706, 7.7194) (81.8706, 7.5249) knots 0 0 0 1 2 2 2
  spline S47 degree 2 poles (81.8706, 7.5249) (81.8706, 7.2501) (81.3961, 6.8403) (81.0097, 6.7807) knots 0 0 0 1 2 2 2
  line L23 (81.0097, 6.7807) -> (81.0097, 6.7496)
  spline S48 degree 2 poles (81.0097, 6.7496) (81.1808, 6.734) (81.505, 6.651) (81.6606, 6.5577) knots 0 0 0 1 2 2 2
  spline S49 degree 2 poles (81.6606, 6.5577) (81.8058, 6.4747) (81.9951, 6.2102) (81.9951, 6.0287) knots 0 0 0 1 2 2 2
  point P0 (0, 0)
  constraints: 2 other
extrude "Выдавливание9" cut sketch "Эскиз12" against normal blind 20
extrude "Выдавливание10" cut sketch "Эскиз14" against normal blind 20
fillet "Сопряжение1" radius 4 2 edges at (0, 22.5, 0) (0, 22.5, 30)
fillet "Сопряжение2" radius 4 4 edges at (150, 5, 30) (150, 5, 0) (150, 35, 30) (150, 35, 0)
fillet "Сопряжение3" radius 4 2 edges at (120, 35, 0) (120, 35, 30)
sketch "Эскиз15" plane through (150, 40, 26) normal (0, 1, 0) x (1, 0, 0)
  circle A0 centre (-15, 11) radius 2 projected
  circle A1 centre (-15, 11) radius 4
  point P0 (-150, 26)
  dimension "d46" = 8
  constraints: 1 centre point, 1 coincident
  measures "d46" diameter of A1
extrude "Выдавливание11" cut sketch "Эскиз15" against normal blind 4.3
fillet "Сопряжение4" radius 4 4 edges at (147.5, 20, 20) (147.5, 20, 10) (122.5, 20, 20) (122.5, 20, 10)
